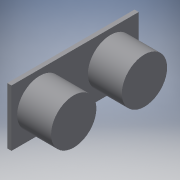
# Autodesk Inventor part: HCSR04
Saved by Autodesk Inventor 2019 (Build 230136000, 136)
## iProperties
Created: 2022-09-15
Part Number: HCSR04
Material: Generic
Document SubType Name: Modeling
Designer: ThinkPad
Density: 0.971583 g/cm^3
Appearance: Default
Mass: 6 g
Surface Area: 32.0137 cm^2
Volume: 6.17549 cm^3
Author: ThinkPad
Autodesk Inventor part; units mm, degrees
ref_plane "YZ Plane" through (0, 0, 0) normal (1, 0, 0) x (0, 1, 0)
ref_plane "XZ Plane" through (0, 0, 0) normal (0, 1, 0) x (-1, 0, 0)
ref_plane "XY Plane" through (0, 0, 0) normal (0, 0, 1) x (1, 0, 0)
sketch "Sketch1" plane through (0, 0, 0) normal (1, 0, 0) x (0, 1, 0)
  line L0 (5.2514, 14.5134) -> (-14.7486, 14.5134)
  line L1 (-14.7486, 14.5134) -> (-14.7486, -30.4866)
  line L2 (-14.7486, -30.4866) -> (5.2514, -30.4866)
  line L3 (5.2514, -30.4866) -> (5.2514, 14.5134)
  line L4 (3.2514, 12.5134) -> (-12.7486, 12.5134)
  line L5 (-12.7486, 12.5134) -> (-12.7486, -28.4866)
  line L6 (-12.7486, -28.4866) -> (3.2514, -28.4866)
  line L7 (3.2514, -28.4866) -> (3.2514, 12.5134)
  circle A0 centre (-4.7486, -20.4866) radius 8
  line L8 (3.2514, -7.9866) -> (-3.9727, -7.9866)
  circle A1 centre (-4.7486, 4.5134) radius 8
  point P0 (0, 0)
  dimension "d0" = 20
  dimension "d1" = 45
  constraints: 18 end point, 4 parallel, 2 centre point, 2 horizontal, 2 perpendicular, 1 midpoint, 1 symmetric about line, 1 tangent, 4 other
  measures "d0" distance of L2.end L1.end
  measures "d1" distance of L1.end L0.end
extrude "Extrusion1" add sketch "Sketch1" along normal blind 1.5 contours L3 L2 L1 L0 | L7 A1 L4 | A1 L5 L4 | A1 | L7 A0 L5 A1 | A0 L6 L5 | A0 | L7 L6 A0
extrude "Extrusion2" add sketch "Sketch1" along normal blind 13.5 contours A1 | A0
body "Solid1"
